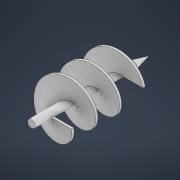
# Autodesk Inventor part: Pieza de practica 8
Saved by Autodesk Inventor 2022 (Build 260153000, 153)
## iProperties
Created: 2022-08-03
Part Number: Pieza de practica 8
Material: Genérico
Document SubType Name: Modeling
Designer: aleon
Density: 1 g/cm^3
Appearance: Valor por defecto
Author: aleon
Autodesk Inventor part; units mm, degrees
ref_plane "YZ Plane" through (0, 0, 0) normal (1, 0, 0) x (0, 1, 0)
ref_plane "XZ Plane" through (0, 0, 0) normal (0, 1, 0) x (-1, 0, 0)
ref_plane "XY Plane" through (0, 0, 0) normal (0, 0, 1) x (1, 0, 0)
sketch "Boceto1" plane through (0, 0, 0) normal (0, 1, 0) x (-1, 0, 0)
  line L0 (0, 0) -> (1.4, 0)
  line L1 (1.4, 0) -> (1.4, -37)
  line L2 (1.4, -37) -> (0, -42.6)
  line L3 (0, -42.6) -> (0, 0)
  dimension "d0" = 1.4
  dimension "d1" = 5.6
  dimension "d2" = 42.6
  constraints: 8 end point, 1 horizontal, 1 parallel, 1 perpendicular
  measures "d0" distance of L0.start L0.end
  measures "d1" vertical distance of L2.end L1.end
  measures "d2" distance from line of L2.end L0
revolve "Revolución1" add sketch "Boceto1" angle 360 about axis through (0, 0, -42.6) along (0, 0, 1)
sketch "Boceto2" plane through (0, 0, 0) normal (0, 1, 0) x (-1, 0, 0)
  line L0 (-1.4, 0) -> (-1.4, -37) projected
  line L1 (-1.4, -5.6) -> (-9, -5.6)
  line L2 (-9, -5.6) -> (-9, -6.4)
  line L3 (-9, -6.4) -> (-1.4, -6.4)
  line L4 (-1.4, -5.6) -> (-1.4, -6.4)
  line L5 (-1.4, 0) -> (1.4, 0) projected
  line L6 (0, 0) -> (0, -42.6)
  line L7 (1.4, -37) -> (0, -42.6) projected
  dimension "d4" = 0.8
  dimension "d5" = 7.6
  dimension "d6" = 5.6
  constraints: 10 end point, 3 perpendicular, 3 point on line, 1 horizontal, 1 vertical
  measures "d4" distance of L1.end L2.end
  measures "d5" distance of L1.start L1.end
  measures "d6" distance between parallel lines of L1 L5
coil "Bobina1" sketch "Boceto2" operation add axis through (0, 0, 0) along (0, 0, -1) pitch 8.6667 turns 3 hand right
